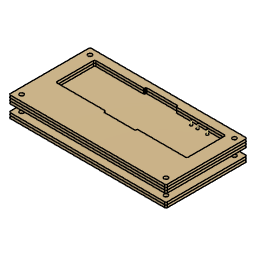
Hanshow Nebular 350-N - Fusion360 (Autodesk Fusion 360 design; units mm, degrees)
Autodesk Fusion 360 part; units mm, degrees
sketch "Skizze1" plane through (0, 0, 0) normal (0, 0, 1) x (1, 0, 0)
  line L0 (-51.7, -14.2) -> (-51.7, 14.4)
  line L1 (51.7, 14.4) -> (51.7, -14.2)
  line L2 (12, -16.7) -> (-12, -16.7)
  line L3 (-12.5, -16.2) -> (-12.5, -15.7)
  line L4 (12.5, -15.7) -> (12.5, -16.2)
  line L5 (-12, 16.9) -> (12, 16.9)
  line L6 (12.5, 16.4) -> (12.5, 15.9)
  line L7 (-12.5, 15.9) -> (-12.5, 16.4)
  line L8 (52.9, 16.9) -> (-52.9, 16.9)
  line L9 (-52.9, 16.9) -> (-52.9, -35.4)
  line L10 (-52.9, -35.4) -> (52.9, -35.4)
  line L11 (52.9, -35.4) -> (52.9, 16.9)
  line L12 (-61, 22) -> (61, 22)
  line L13 (62, 21) -> (62, -41)
  line L14 (61, -42) -> (-61, -42)
  line L15 (-62, -41) -> (-62, 21)
  circle A0 centre (-57, 17) radius 1.6
  circle A1 centre (57, 17) radius 1.6
  circle A2 centre (-57, -37) radius 1.6
  circle A3 centre (57, -37) radius 1.6
  circle A4 centre (39.6, 13) radius 1
  circle A5 centre (31.98, 13) radius 1
  circle A6 centre (26.9, 13) radius 1
  arc A7 (-61, 22) -> (-62, 21) centre (-61, 21) ccw
  arc A8 (62, 21) -> (61, 22) centre (61, 21) ccw
  arc A9 (-62, -41) -> (-61, -42) centre (-61, -41) ccw
  arc A10 (61, -42) -> (62, -41) centre (61, -41) ccw
  arc A11 (-50.7, 15.4) -> (-51.7, 14.4) centre (-50.7, 14.4) ccw
  arc A12 (-51.7, -14.2) -> (-50.6986, -15.2) centre (-50.7, -14.2) ccw
  arc A13 (51.7, 14.4) -> (50.7, 15.4) centre (50.7, 14.4) ccw
  arc A14 (50.7, -15.2) -> (51.7, -14.2) centre (50.7, -14.2) ccw
  line L16 (-50.7, 15.4) -> (-13, 15.4)
  line L17 (13, 15.4) -> (50.7, 15.4)
  line L18 (50.7, -15.2) -> (13, -15.2)
  line L19 (-13, -15.2) -> (-50.6986, -15.2)
  arc A15 (-13, 15.4) -> (-12.5, 15.9) centre (-13, 15.9) ccw
  arc A16 (12.5, 15.9) -> (13, 15.4) centre (13, 15.9) ccw
  arc A17 (12.5, 16.4) -> (12, 16.9) centre (12, 16.4) ccw
  arc A18 (-12, 16.9) -> (-12.5, 16.4) centre (-12, 16.4) ccw
  arc A19 (-12.5, -15.7) -> (-13, -15.2) centre (-13, -15.7) ccw
  arc A20 (13, -15.2) -> (12.5, -15.7) centre (13, -15.7) ccw
  arc A21 (-12.5, -16.2) -> (-12, -16.7) centre (-12, -16.2) ccw
  arc A22 (12, -16.7) -> (12.5, -16.2) centre (12, -16.2) ccw
  circle A23 centre (26.9, 13) radius 0.45
  circle A24 centre (31.98, 13) radius 0.45
  circle A25 centre (39.6, 13) radius 0.45
  point P0 (-51.7, -15.2)
  point P1 (-51.7, 15.4)
  point P2 (51.7, 15.4)
  point P3 (-12.5, -16.7)
  point P4 (-12.5, -15.2)
  point P5 (12.5, -15.2)
  point P6 (0, -16.15)
  point P7 (12.5, 16.9)
  point P8 (-12.5, 15.4)
  point P9 (-12.5, 16.9)
  point P10 (0, -9.25)
  dimension "d5" = 25
  dimension "d6" = 1.5
  dimension "d7" = 25
  dimension "d8" = 1.5
  dimension "d9" = 105.8
  dimension "d10" = 52.3
  dimension "d17" = 3.2
  dimension "d19" = 3.2
  dimension "d20" = 3.2
  dimension "d21" = 3.2
  dimension "d43" = 2
  dimension "d46" = 2
  dimension "d48" = 2
  dimension "d49" = 1
  dimension "d50" = 1
  dimension "d51" = 1
  dimension "d52" = 1
  dimension "d53" = 1
  dimension "d54" = 1
  dimension "d55" = 1
  dimension "d56" = 1
  dimension "d57" = 0.5
  dimension "d58" = 0.5
  dimension "d59" = 0.5
  dimension "d60" = 0.5
  dimension "d61" = 0.5
  dimension "d62" = 0.5
  dimension "d63" = 0.5
  dimension "d64" = 0.5
  dimension "d73" = 0.9
  dimension "d74" = 0.9
  dimension "d75" = 0.9
  constraint horizontal L18
  constraint perpendicular L0 L18
  constraint parallel L16 L18
  constraint parallel L0 L1
  constraint horizontal L2
  constraint perpendicular L2 L3
  constraint parallel L3 L4
  constraint parallel L6 L7
  constraint horizontal L8
  constraint perpendicular L8 L9
  constraint parallel L8 L10
  constraint parallel L9 L11
  constraint horizontal L12
  constraint vertical L13
  constraint horizontal L14
  constraint vertical L15
  constraint tangent L12 A7
  constraint tangent L15 A7
  constraint tangent L12 A8
  constraint tangent L13 A8
  constraint tangent L14 A9
  constraint tangent L15 A9
  constraint tangent L13 A10
  constraint tangent L14 A10
  constraint coincident P1 L0
  constraint coincident P1 L16
  constraint tangent L0 A11
  constraint tangent A11 L16
  constraint coincident P0 L18
  constraint coincident P0 L0
  constraint tangent A12 L18
  constraint tangent L0 A12
  constraint coincident P2 L16
  constraint coincident P2 L1
  constraint tangent A13 L16
  constraint tangent L1 A13
  constraint tangent A14 L18
  constraint tangent L1 A14
  constraint collinear L16 L17
  constraint collinear L18 L19
  constraint coincident P8 L7
  constraint coincident P8 L16
  constraint tangent L7 A15
  constraint tangent L16 A15
  constraint tangent L6 A16
  constraint tangent L17 A16
  constraint coincident P7 L5
  constraint coincident P7 L6
  constraint tangent L5 A17
  constraint tangent L6 A17
  constraint coincident P9 L5
  constraint coincident P9 L7
  constraint tangent L5 A18
  constraint tangent L7 A18
  constraint coincident P4 L3
  constraint coincident P4 L19
  constraint tangent L3 A19
  constraint tangent L19 A19
  constraint coincident P5 L4
  constraint coincident P5 L18
  constraint tangent L4 A20
  constraint tangent L18 A20
  constraint coincident P3 L2
  constraint coincident P3 L3
  constraint tangent L2 A21
  constraint tangent L3 A21
  constraint tangent L2 A22
  constraint tangent L4 A22
  constraint concentric A6 A23
  constraint concentric A5 A24
  constraint concentric A4 A25
  measures "d5" distance of P4 P5
  measures "d6" distance of P3 P4
  measures "d7" distance of P7 P9
  measures "d8" distance of P8 P9
  measures "d9" distance of L9.end L10.end
  measures "d10" distance of L8.end L9.end
  measures "d17" diameter of A0
  measures "d19" diameter of A1
  measures "d20" diameter of A2
  measures "d21" diameter of A3
  measures "d43" diameter of A4
  measures "d46" diameter of A5
  measures "d48" diameter of A6
  measures "d49" radius of A7
  measures "d50" radius of A8
  measures "d51" radius of A9
  measures "d52" radius of A10
  measures "d53" radius of A11
  measures "d54" radius of A12
  measures "d55" radius of A13
  measures "d56" radius of A14
  measures "d57" radius of A15
  measures "d58" radius of A16
  measures "d59" radius of A17
  measures "d60" radius of A18
  measures "d61" radius of A19
  measures "d62" radius of A20
  measures "d63" radius of A21
  measures "d64" radius of A22
  measures "d73" diameter of A23
  measures "d74" diameter of A24
  measures "d75" diameter of A25
extrude "Extrusion16" add sketch "Skizze1" along normal blind 2 contours L0 L1 L2 L3 L4 L6 L7 L8 L9 L10 L11 A11 A12 A13 A14 L16 L17 L18 L19 A15 A16 A17 A18 A19 A20 A21 A22 | L0 L1 L2 L3 L4 L5 L6 L7 L8 A11 A12 A13 A14 L16 L17 L18 L19 A15 A16 A17 A18 A19 A20 A21 A22 | L12 L13 L14 L15 A7 A8 A9 A10 | A4 | A5 | A6 | A23 | A24 | A25 makes body 1
extrude "Extrusion17" add sketch "Skizze1" along normal blind 2 separate body contours L0 L1 L2 L3 L4 L6 L7 L8 L9 L10 L11 A11 A12 A13 A14 L16 L17 L18 L19 A15 A16 A17 A18 A19 A20 A21 A22 | L0 L1 L2 L3 L4 L5 L6 L7 L8 A11 A12 A13 A14 L16 L17 L18 L19 A15 A16 A17 A18 A19 A20 A21 A22 | L12 L13 L14 L15 A7 A8 A9 A10 | A4 | A5 | A6 makes body 2
move_body "Verschieben3" bodies 2 to x (1, 0, 0) y (0, 1, 0) z (0, 0, 1) at (0, 0, 2)
extrude "Extrusion18" add sketch "Skizze1" along normal blind 2 separate body contours L0 L1 L2 L3 L4 L6 L7 L8 L9 L10 L11 A11 A12 A13 A14 L16 L17 L18 L19 A15 A16 A17 A18 A19 A20 A21 A22 | L0 L1 L2 L3 L4 L5 L6 L7 L8 A11 A12 A13 A14 L16 L17 L18 L19 A15 A16 A17 A18 A19 A20 A21 A22 | L12 L13 L14 L15 A7 A8 A9 A10 makes body 3
move_body "Verschieben4" bodies 3 to x (1, 0, 0) y (0, 1, 0) z (0, 0, 1) at (0, 0, 10)
extrude "Extrusion19" add sketch "Skizze1" along normal blind 2 separate body contours L0 L1 L2 L3 L4 L6 L7 L8 L9 L10 L11 A11 A12 A13 A14 L16 L17 L18 L19 A15 A16 A17 A18 A19 A20 A21 A22 | L12 L13 L14 L15 A7 A8 A9 A10 makes body 4
move_body "Verschieben5" bodies 4 to x (1, 0, 0) y (0, 1, 0) z (0, 0, 1) at (0, 0, 12)
copy_body "Körper kopieren/einfügen1" bodies 4 makes body 5
move_body "Verschieben6" bodies 5 to x (1, 0, 0) y (0, 1, 0) z (0, 0, 1) at (0, 0, 2)
extrude "Extrusion20" add sketch "Skizze1" along normal blind 14 separate body contours A23 | A24 | A25 makes body 6 at (27.0851, 13.4102, 9.3333) makes body 7 at (32.1651, 13.4102, 9.3333) makes body 8 at (39.1853, 12.8252, 9.3333)
move_body "Verschieben8" bodies 6 7 8 to x (1, 0, 0) y (0, 1, 0) z (0, 0, 1) at (0, 0, 2)
chamfer "Fase1" distance 0.3 angle 45 3 edges at (26.4805, 12.8373, 16) (31.5605, 12.8373, 16) (39.1805, 12.8373, 16) on bodies 6 7 8
move_body "Verschieben7" [rolled back]
named bodies: "Layer 0", "Layer 1", "Layer 2", "Layer 3", "Layer 4", "Pin GND", "Pin TX", "Pin RST"
